Autodesk Fusion 360 part; units mm, degrees
note: some values were not read from the file. Set by a fixed rule: which sketch regions a step uses.
(part 2 of 2)
equation "d119 = finger_height + 1 mm"
equation "d120 = finger_base"
equation "d121 = finger_height + 1 mm"
equation "d122 = finger_base"
equation "d123 = finger_height + 1 mm"
equation "d124 = finger_base"
equation "d125 = Thickness"
equation "d127 = Thickness"
equation "d128 = divider_width"
equation "d131 = finger_base"
equation "d132 = finger_height"
equation "d133 = finger_base"
equation "d134 = finger_height"
equation "d135 = finger_base"
equation "d136 = finger_height"
equation "d137 = finger_base"
equation "d138 = finger_height"
equation "d139 = divider_width"
equation "d141 = -Thickness"
equation "d151 = -Thickness"
equation "d155 = Thickness"
equation "d163 = -Thickness"
equation "d166 = finger_base"
equation "d168 = finger_base"
equation "d169 = -Thickness"
equation "d177 = Thickness"
equation "d179 = finger_base"
equation "d181 = finger_base"
equation "d184 = Thickness"
equation "d186 = Base"
equation "d188 = Thickness"
equation "d190 = Base"
equation "d192 = Thickness"
equation "d194 = finger_base"
equation "d195 = finger_height"
named bodies: "front", "base", "top", "back", "left", "supporting 1", "supporting 2_delete", "divider_delete", "supporting 3_delete", "supporting 4", "motor holder", "right", "divider", "supporting 2", "supporting 3"
